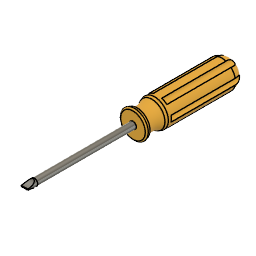
14_DAY- Screwdriver (Autodesk Fusion 360 design; units mm, degrees)
part number: 2026-01-01-10-49-18-154
part number: 2026-01-01-11-35-02-095
part number: 2026-01-01-11-35-25-743
part number: 2026-01-01-13-23-50-895
Autodesk Fusion 360 part; units mm, degrees
sketch "Sketch1" plane through (0, 0, 0) normal (0, 0, 1) x (1, 0, 0) in component "Handle"
  circle A0 centre (0, 0) radius 14
  dimension "d1" = 28
  constraint coincident A0.centre origin
  measures "d1" diameter of A0
extrude "Extrude1" add sketch "Sketch1" against normal blind 100 makes body 1 in component "Handle"
sketch "Sketch2" plane through (0, 0, -100) normal (0, 0, -1) x (-1, 0, 0) in component "Handle"
  circle A0 centre (0, 0) radius 14
  circle A1 centre (-14, 0) radius 3
  dimension "d4" = 6
  constraint coincident A0 A1.centre
  constraint horizontal A0.centre A1.centre
  measures "d4" diameter of A1
extrude "Extrude2" cut sketch "Sketch2" against normal blind 75 contours A0 A1 picked at (-12.9761, 0) bodies 1 in component "Handle"
pattern_circular "C-Pattern1" count 6 over 360 about axis through (0, 0, 1.75) along (0, 0, 1) of "Extrude2" in component "Handle"
sketch "Sketch3" plane through (0, 0, 0) normal (1, 0, 0) x (0, 0, -1) in component "Handle"
  line L0 (0, -14) -> (100, -14)
  line L1 (100, 14) -> (0, 14)
  arc A0 (3, 14) -> (20.3205, 14) centre (11.6603, 25) ccw
  dimension "d9" = 3
  dimension "d10" = 11
  dimension "d11" = 14
  constraint coincident L1 A0.end
  constraint coincident L1 A0.start
  measures "d9" distance of L1.end A0.start
  measures "d10" vertical distance of L1.end A0.centre
  measures "d11" radius of A0
revolve "Revolve1" cut sketch "Sketch3" angle 360 about axis through (0, 0, 1.75) along (0, 0, 1) bodies 1 in component "Handle"
sketch "Sketch4" plane through (0, 0, 0) normal (0, 0, 1) x (1, 0, 0) in component "Handle"
  circle A0 centre (0, 0) radius 14
  circle A1 centre (0, 0) radius 3.5
  dimension "d13" = 7
  constraint coincident A0.centre A1.centre
  measures "d13" diameter of A1
extrude "Extrude3" cut sketch "Sketch4" against normal blind 50 contours A1 bodies 1 in component "Handle"
fillet "Fillet1" radius 5 2 edges at (-13.0526, -5.0626, -3) (-13.0526, 5.0626, -20.3205) on bodies 1 in component "Handle"
fillet "Fillet1" radius 1.5 1 edges at (-13.0526, -5.0626, 0) on bodies 1 in component "Handle"
fillet "Fillet1" radius 10 6 edges at (0, 14, -100) (12.1244, 7, -100) (12.1244, -7, -100) (0, -14, -100) (-12.1244, -7, -100) (-12.1244, 7, -100) on bodies 1 in component "Handle"
sketch "Sketch1 (2)" plane through (-0.2425, 2.53, -50) normal (0, 0, 1) x (1, 0, 0) in component "Shank"
  circle A0 centre (0.2425, -2.53) radius 3.5
  circle A1 centre (0.2425, -2.53) radius 3.5
  constraint concentric A0 A1
extrude "Extrude1'" add sketch "Sketch1 (2)" along normal blind 150 separate body makes body 2 in component "Shank"
extrude "Extrude1''" add 1 faces at (0.8715, -1.0104, 100) along direction (0, 0, 1) blind 10 separate body on bodies 2 makes body 3 in component "Tip"
sketch "Sketch1 (3)" plane through (0, 0, 0) normal (1, 0, 0) x (0, 0, -1) in component "Tip"
  line L0 (-100, 3.5) -> (-110, 3.5)
  line L1 (-110, -3.5) -> (-100, -3.5)
  arc A0 (-110, 0.5) -> (-101, 3.5) centre (-110.3322, 16.4966) ccw
  line L2 (-110, 3.5) -> (-110, 0.5)
  line L3 (-110, 3.5) -> (-101, 3.5)
  point P0 (-110, 0)
  dimension "d26" = 0.5
  dimension "d27" = 9
  dimension "d28" = 16
  constraint coincident L0 A0.end
  constraint vertical L0.end A0.start
  constraint coincident L0.end L2.start
  measures "d26" vertical distance of A0.start P0
  measures "d27" distance of L0.end A0.end
  measures "d28" distance of A0.end A0.centre
extrude "Extrude2'" cut sketch "Sketch1 (3)" along normal through all and the other way through all bodies 3 in component "Tip"
mirror "Mirror1" about plane through (0, 0, 0) normal (0, 1, 0) of "Extrude2'" in component "Tip"
component "Shank" placed x (1, 0, 0) y (0, 1, 0) z (0, 0, 1) at (0, 0, 0)
component "Handle" placed x (1, 0, 0) y (0, 1, 0) z (0, 0, 1) at (0, 0, 0)
component "Tip" placed x (1, 0, 0) y (0, 1, 0) z (0, 0, 1) at (0, 0, 0)
